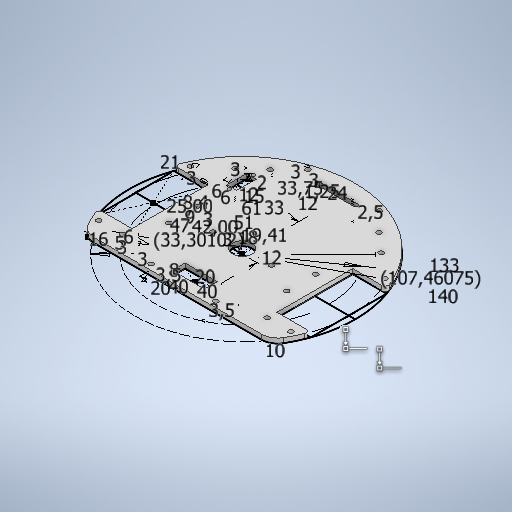
# Autodesk Inventor part: base_chasis_v5
Saved by Autodesk Inventor 2025.2 (Build 292293000, 293)
## iProperties
Created: 2025-03-12
Part Number: base_chasis_v5
Material: Generic
Document SubType Name: Modeling
Designer: cdavi
Density: 1 g/cm^3
Appearance: Default
Author: cdavi
Autodesk Inventor part; units mm, degrees
ref_plane "YZ Plane" through (0, 0, 0) normal (1, 0, 0) x (0, 1, 0)
ref_plane "XZ Plane" through (0, 0, 0) normal (0, 1, 0) x (-1, 0, 0)
ref_plane "XY Plane" through (0, 0, 0) normal (0, 0, 1) x (1, 0, 0)
sketch "Sketch1" plane through (0, 0, 0) normal (0, 1, 0) x (-1, 0, 0)
  line L0 (51.9615, 40) -> (-51.9615, 40)
  line L1 (12, -59.7203) -> (-12, -59.7203)
  line L2 (-12, -57.2203) -> (12, -57.2203)
  circle A0 centre (0, 0) radius 6
  circle A1 centre (-22.1, -62.7203) radius 1.5
  circle A2 centre (-44.9077, 29.5) radius 1.5
  circle A3 centre (-60.2695, -28.1041) radius 1.5
  circle A4 centre (60.2695, -28.1041) radius 1.5
  circle A5 centre (-20, 36.5) radius 1.5
  circle A6 centre (44.9077, 29.5) radius 1.5
  circle A7 centre (20, 36.5) radius 1.5
  circle A8 centre (22.1, -62.7203) radius 1.5
  arc A9 (12, -59.7203) -> (12, -57.2203) centre (12, -58.4703) ccw
  arc A10 (-12, -57.2203) -> (-12, -59.7203) centre (-12, -58.4703) ccw
  circle A11 centre (0, 0) radius 66.5 construction
  circle A12 centre (0, 0) radius 53.7304 construction
  line L3 (0, 0) -> (0, 40)
  arc A13 (-60.6218, 35) -> (60.6218, 35) centre (0, 0) ccw
  arc A14 (-51.9615, 40) -> (-60.6218, 35) centre (-51.9615, 30) ccw
  arc A15 (60.6218, 35) -> (51.9615, 40) centre (51.9615, 30) ccw
  line L4 (0, 0) -> (-70, 0)
  line L5 (0, 0) -> (60.2695, -28.1041) construction
  line L6 (0, 0) -> (66.5, 0)
  line L7 (0, 0) -> (44.9077, 29.5) construction
  line L8 (44.9375, 23.5) -> (65.9375, 23.5)
  line L9 (65.9375, 23.5) -> (65.9375, -23.5)
  line L10 (65.9375, -23.5) -> (44.9375, -23.5)
  line L11 (44.9375, -23.5) -> (44.9375, 23.5)
  line L12 (44.9375, 23.5) -> (65.9375, -23.5) construction
  line L13 (65.9375, 23.5) -> (44.9375, -23.5) construction
  circle A16 centre (36.5375, -9) radius 1.5
  circle A17 centre (36.5375, 9) radius 1.5
  circle A18 centre (18, 0) radius 1.5
  circle A19 centre (33.75, -51) radius 1.5
  circle A20 centre (-18, 0) radius 1.5
  circle A21 centre (-33.75, -51) radius 1.5
  line L14 (-44.9375, 23.5) -> (-65.9375, 23.5)
  line L15 (-65.9375, 23.5) -> (-65.9375, -23.5)
  line L16 (-65.9375, -23.5) -> (-44.9375, -23.5)
  line L17 (-44.9375, -23.5) -> (-44.9375, 23.5)
  circle A22 centre (-36.5375, -9) radius 1.5
  circle A23 centre (-36.5375, 9) radius 1.5
  line L18 (10, 33.5) -> (-10, 33.5)
  line L19 (-10, 33.5) -> (-10, 25.5)
  line L20 (-10, 25.5) -> (10, 25.5)
  line L21 (10, 25.5) -> (10, 33.5)
  line L22 (10, 33.5) -> (-10, 25.5) construction
  line L23 (-10, 33.5) -> (10, 25.5) construction
  line L24 (39, -29.5) -> (33, -29.5)
  line L25 (33, -29.5) -> (33, -41.5)
  line L26 (33, -41.5) -> (39, -41.5)
  line L27 (39, -41.5) -> (39, -29.5)
  circle A24 centre (36, -43) radius 1
  line L28 (39, -35.5) -> (33, -35.5)
  circle A25 centre (36, -28) radius 1
  circle A26 centre (45.3318, -40.817) radius 1.5
  circle A27 centre (-44.9077, 29.5) radius 1.5
  circle A28 centre (-45.3318, -40.817) radius 1.5
  line L29 (44.9077, 29.5) -> (44.9077, 34.5)
  line L30 (44.9077, 34.5) -> (60.9077, 34.5)
  line L31 (0, 0) -> (22.1, -62.7203) construction
  circle A29 centre (59.5987, 29.5) radius 1.5
  circle A30 centre (-59.5987, 29.5) radius 1.5
  line L32 (45.3318, -40.817) -> (0, 0) construction
  point P0 (-5.9883, -61.0615)
  point P1 (55.4375, 0)
  point P2 (-65.9375, -23.5)
  point P3 (0, 29.5)
  point P4 (36, -41.5)
  point P5 (56.9615, 38.6603)
  point P6 (0, -6)
  dimension "d12" = 12
  dimension "d0" = 3
  dimension "d1" = 3
  dimension "d4" = 3
  dimension "d15" = 24
  dimension "d16" = 3
  dimension "d62" = 2.5
  dimension "d148" = 3.5
  dimension "d151" = 3
  dimension "d182" = 1.25
  dimension "d276" = 133
  dimension "d285" = 140
  dimension "d286" = 40
  dimension "d287" = 10
  dimension "d288" = 12
  dimension "d289" = 40
  dimension "d290" = 3.5
  dimension "d291" = 20
  dimension "d293" = 25
  dimension "d300" = 21
  dimension "d301" = 47
  dimension "d304" = 3
  dimension "d305" = 8.4
  dimension "d306" = 9
  dimension "d307" = 3
  dimension "d311" = 18
  dimension "d317" = 51
  dimension "d318" = 33.75
  dimension "d321" = 20
  dimension "d322" = 8
  dimension "d323" = 12
  dimension "d324" = 6
  dimension "d325" = 6
  dimension "d326" = 2
  dimension "d327" = 15
  dimension "d338" = 33
  dimension "d342" = 5
  dimension "d344" = 16
  dimension "d345" = 6
  dimension "d346" = 33.301
  dimension "d347" = 107.4608
  dimension "d348" = 19.41
  dimension "d350" = 61
  dimension "d351" = 42
  dimension "d352" = 3
  constraints: 67 end point, 30 centre point, 22 point on circle, 14 symmetric about line, 9 midpoint, 8 horizontal, 7 parallel, 6 coincident, 5 perpendicular, 4 point on line, 4 tangent, 3 equal radius, 3 vertical alignment, 2 horizontal alignment, 2 vertical, 15 other
  measures "d0" diameter of A6
  measures "d1" diameter of A7
  measures "d4" diameter of A4
  measures "d15" distance of L1.end L1.start
  measures "d16" diameter of A8
  measures "d62" distance between parallel lines of L1 L2
  measures "d148" distance from line of L0 A7.centre
  measures "d151" vertical distance of L1.start L31.end
  measures "d182" distance of point (12, -58.47) L1.start
  measures "d276" diameter of A11
  measures "d285" diameter of A13
  measures "d286" distance from line of L0 point (0, 0)
  measures "d287" radius of A14
  measures "d288" horizontal distance of point (0, 0) A9.centre
  measures "d289" distance of A7.centre A5.centre
  measures "d290" distance from line of L0 A5.centre
  measures "d291" distance from line of L3 A7.centre
  measures "d293" angle of L6 L5
  measures "d300" distance of L9.end L10.end
  measures "d301" distance of L10.end L8.start
  measures "d304" diameter of A16
  measures "d305" distance from line of L11 A16.centre
  measures "d306" distance from line of L6 A16.centre
  measures "d307" diameter of A18
  measures "d311" distance of point (0, 0) A18.centre
  measures "d317" vertical distance of A18.centre A19.centre
  measures "d318" distance from line of L3 A19.centre
  measures "d321" distance of L19.end L20.end
  measures "d322" distance between parallel lines of L18 L20
  measures "d323" distance of L24.end L25.end
  measures "d324" distance of L24.start L24.end
  measures "d325" distance from line of L10.end L24
  measures "d326" diameter of A24
  measures "d327" distance of A25.centre A24.centre
  measures "d338" distance between parallel lines of L3 L25
  measures "d342" distance of L7.end L29.end
  measures "d344" distance of L29.end L30.end
  measures "d345" distance from line of L8 L7.end
  measures "d346" angle of L6 L7
  measures "d347" diameter of A12
  measures "d348" angle of L3 L31
  measures "d350" distance of L32.start L4.start
  measures "d351" angle of L6 L32
  measures "d352" diameter of A26
extrude "Extrusion1" add sketch "Sketch1" along normal blind 3 contours A15 A13 L8 L11 L6 A18 A0 L3 L20 L21 L18 L0 | L3 L18 L19 L20 A0 L4 A20 L17 L14 A13 A14 L0 | A13 L16 L17 L4 A20 A0 L6 A18 L11 L10
fillet "Fillet1" radius 2 1 edges at (65.9375, 1.5, 23.5)
fillet "Fillet2" radius 2 3 edges at (65.9375, 1.5, -23.5) (-65.9375, 1.5, -23.5) (-65.9375, 1.5, 23.5)
body "Solid1"
